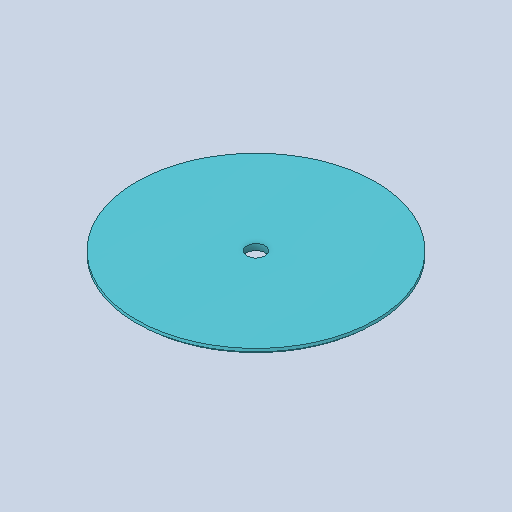
# Autodesk Inventor part: TorsOsc-202511-cell-plate
Saved by Autodesk Inventor 2026 (Build 300175050, 175E)
## iProperties
Created: 2025-12-02
Part Number: TorsOsc-202511-cell-plate
Material: Epoxy Resin
Document SubType Name: Modeling
Designer: schanen
Density: 1.14 g/cm^3
Appearance: Cadet Blue
Mass: 1.63522 g
Surface Area: 26.1355 cm^2
Volume: 1.24826 cm^3
Author: schanen
Autodesk Inventor part; units mm, degrees
ref_plane "YZ Plane" through (0, 0, 0) normal (1, 0, 0) x (0, 1, 0)
ref_plane "XZ Plane" through (0, 0, 0) normal (0, 1, 0) x (-1, 0, 0)
ref_plane "XY Plane" through (0, 0, 0) normal (0, 0, 1) x (1, 0, 0)
sketch "Sketch1" plane through (0, 0, 0) normal (1, 0, 0) x (0, 1, 0)
  line L0 (1, 1.5) -> (0, 1.5)
  line L1 (1, 20) -> (1, 1.5)
  line L2 (-0.2, 0) -> (1.2, 0) projected
  line L3 (1, 20) -> (0.5, 20)
  line L4 (0.5, 20) -> (0.5, 19.45)
  line L5 (0, 19.45) -> (0, 1.5)
  line L6 (1, 20) -> (1, 20)
  line L7 (1, 20) -> (1, 19)
  line L8 (1, 19) -> (1, 19)
  line L9 (1, 19) -> (1, 20)
  line L10 (0.5, 19.45) -> (0, 19.45)
  point P0 (0, 0)
  point P1 (1, 19)
  dimension "d1" = 1.5
  dimension "d14" = 20
  dimension "d15" = 0.55
  dimension "d16" = 1
  dimension "d17" = 0.5
  dimension "d18" = 0
  dimension "d20" = 1
  constraints: 20 end point, 4 perpendicular, 3 horizontal, 1 collinear, 1 vertical alignment
  measures "d1" distance between parallel lines of L2 L0
  measures "d14" distance between parallel lines of L2 L3
  measures "d15" distance of L3.end L4.end
  measures "d16" distance between parallel lines of L5 L1
  measures "d17" distance of L1.start L3.end
  measures "d18" distance of L7.end L8.end
  measures "d20" distance of L6.end L7.end
revolve "Revolution1" add sketch "Sketch1" angle 360 about axis through (0, -10, 0) along (0, 1, 0)
sketch "Sketch4" plane through (0, 0, 0) normal (0, -1, 0) x (1, 0, 0)
  circle A0 centre (18.5, 0) radius 0.5
  circle A1 centre (0, 0) radius 19.45 projected
  dimension "d21" = 1
  dimension "d22" = 18.5
  constraints: 1 centre point
  measures "d21" diameter of A0
  measures "d22" distance of A1.centre A0.centre
extrude "Extrusion1" add sketch "Sketch4" along normal blind 1 draft -45 contours A0
pattern_circular "Circular Pattern1" count 36 over 360 about axis through (0, 0.75, 0) along (0, 1, 0) of "Extrusion1"
body "Solid1"
